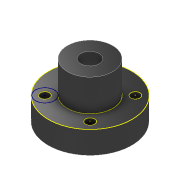
# Autodesk Inventor part: perilla
Saved by Autodesk Inventor 2022 (Build 260153000, 153)
## iProperties
Created: 2022-11-14
Part Number: perilla
Material: Generic
Document SubType Name: Modeling
Designer: ferna
Density: 1 g/cm^3
Appearance: Glossy - Black
Author: ferna
Autodesk Inventor part; units mm, degrees
ref_plane "YZ Plane" through (0, 0, 0) normal (1, 0, 0) x (0, 1, 0)
ref_plane "XZ Plane" through (0, 0, 0) normal (0, 1, 0) x (-1, 0, 0)
ref_plane "XY Plane" through (0, 0, 0) normal (0, 0, 1) x (1, 0, 0)
sketch "Sketch1" plane through (0, 0, 0) normal (0, 1, 0) x (-1, 0, 0)
  circle A0 centre (0, 0) radius 18.4566
  circle A1 centre (10, 10) radius 2
  circle A2 centre (10, -10) radius 2
  circle A3 centre (-10, -10) radius 2
  circle A4 centre (-10, 10) radius 2
  point P0 (8.8496, 0)
  constraints: 5 centre point
extrude "Extrusion1" add sketch "Sketch1" along normal blind 10
sketch "Sketch2" plane through (0, 10, 0) normal (0, 1, 0) x (1, 0, 0)
  circle A0 centre (0, 0) radius 10
  dimension "d2" = 20
  constraints: 1 centre point, 1 coincident
  measures "d2" diameter of A0
extrude "Extrusion2" add sketch "Sketch2" along normal blind 14
sketch "Sketch3" plane through (0, 24, 0) normal (0, 1, 0) x (1, 0, 0)
  circle A0 centre (0, 0) radius 4
  dimension "d5" = 8
  constraints: 1 centre point, 1 coincident
  measures "d5" diameter of A0
extrude "Extrusion3" cut sketch "Sketch3" against normal blind 14
sketch "Sketch4" plane through (0, 0, 0) normal (1, 0, 0) x (0, 1, 0)
  line L0 (24, -10) -> (24, 10) projected
  line L1 (24, 0) -> (17, 0)
  circle A0 centre (17, 0) radius 2
  point P0 (0, 0)
  dimension "d8" = 7
  dimension "d9" = 4
  constraints: 2 end point, 1 centre point, 1 coincident, 1 horizontal, 1 midpoint
  measures "d8" distance of L1.start L1.end
  measures "d9" diameter of A0
extrude "Extrusion4" cut sketch "Sketch4" against normal blind 14
sketch "Sketch5" plane through (0, 10, 0) normal (0, 1, 0) x (1, 0, 0)
  circle A0 centre (0, 0) radius 10 projected
  circle A1 centre (0, 0) radius 18.4566 projected
  circle A2 centre (10, -10) radius 2 projected
  circle A3 centre (10, 10) radius 2 projected
  circle A4 centre (-10, 10) radius 2 projected
  circle A5 centre (-10, -10) radius 2 projected
  circle A6 centre (-10, -10) radius 2 projected
  circle A7 centre (-10, -10) radius 4.1421
  circle A8 centre (0, 0) radius 10 projected
  circle A9 centre (-10, 10) radius 2 projected
  circle A10 centre (-10, 10) radius 4.1421
  constraints: 2 centre point, 2 coincident, 2 tangent
body "Solid1"
